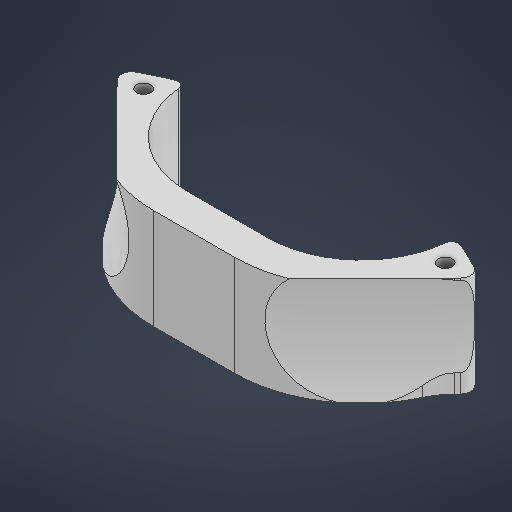
# Autodesk Inventor part: Ballkuhle
Saved by Autodesk Inventor 2025.3 (Build 293356000, 356)
## iProperties
Created: 2024-10-04
Part Number: Ballkuhle
Material: Generisch
Document SubType Name: Modeling
Designer: Mathimazierer
Density: 1 g/cm^3
Appearance: Vorgabe
Author: Mathimazierer
Autodesk Inventor part; units mm, degrees
ref_plane "YZ Plane" through (0, 0, 0) normal (1, 0, 0) x (0, 1, 0)
ref_plane "XZ Plane" through (0, 0, 0) normal (0, 1, 0) x (-1, 0, 0)
ref_plane "XY Plane" through (0, 0, 0) normal (0, 0, 1) x (1, 0, 0)
sketch "Skizze6" plane through (0, 0, 0) normal (0, 0, 1) x (1, 0, 0)
  arc A0 (21.4454, -27.1023) -> (20.0312, -26.5165) centre (20.0312, -28.5165) ccw
  line L0 (20.0312, -26.5165) -> (-20.0312, -26.5165)
  arc A1 (-20.0312, -26.5165) -> (-21.4454, -27.1023) centre (-20.0312, -28.5165) ccw
  line L1 (-21.4454, -27.1023) -> (-51.9723, -57.6292)
  line L2 (-51.9723, -57.6292) -> (-42.4264, -67.1751)
  arc A2 (-38.3776, -89.6293) -> (-42.4264, -67.1751) centre (-56.5685, -81.3173) ccw
  arc A3 (-38.3776, -89.6293) -> (38.3776, -89.6293) centre (0, 0) ccw
  arc A4 (42.4264, -67.1751) -> (38.3776, -89.6293) centre (56.5685, -81.3173) ccw
  line L3 (42.4264, -67.1751) -> (51.9724, -57.6292)
  line L4 (51.9724, -57.6292) -> (21.4454, -27.1023)
  circle A5 centre (37.8302, -37.8302) radius 1.65
  circle A6 centre (37.8302, 37.8302) radius 1.65
  circle A7 centre (-37.8302, -37.8302) radius 1.65
  circle A8 centre (-37.8302, 37.8302) radius 1.65
  circle A9 centre (-22.7665, 22.7665) radius 1.6
  circle A10 centre (22.7665, 22.7665) radius 1.6
  circle A11 centre (22.7665, -22.7665) radius 1.6
  circle A12 centre (-22.7665, -22.7665) radius 1.6
  line L5 (19.0165, -19.0165) -> (19.0165, 19.0165)
  line L6 (19.0165, 19.0165) -> (-19.0165, 19.0165)
  line L7 (-19.0165, 19.0165) -> (-19.0165, -19.0165)
  line L8 (-19.0165, -19.0165) -> (19.0165, -19.0165)
  line L9 (26.5165, -20.8596) -> (57.6292, -51.9723)
  line L10 (57.6292, -51.9723) -> (67.1751, -42.4264)
  arc A13 (89.6293, -38.3776) -> (67.1751, -42.4264) centre (81.3173, -56.5685) ccw
  arc A14 (89.6293, -38.3776) -> (89.6293, 38.3776) centre (0, 0) ccw
  arc A15 (67.1751, 42.4264) -> (89.6293, 38.3776) centre (81.3173, 56.5685) ccw
  line L11 (67.1751, 42.4264) -> (57.6292, 51.9724)
  line L12 (57.6292, 51.9724) -> (26.5165, 20.8597)
  line L13 (26.5165, 20.8597) -> (26.5165, -20.8596)
  line L14 (-26.5165, 20.8596) -> (-57.6292, 51.9723)
  line L15 (-57.6292, 51.9723) -> (-67.1751, 42.4264)
  arc A16 (-89.6293, 38.3776) -> (-67.1751, 42.4264) centre (-81.3173, 56.5685) ccw
  arc A17 (-89.6293, 38.3776) -> (-89.6293, -38.3776) centre (0, 0) ccw
  arc A18 (-67.1751, -42.4264) -> (-89.6293, -38.3776) centre (-81.3173, -56.5685) ccw
  line L16 (-67.1751, -42.4264) -> (-57.6292, -51.9724)
  line L17 (-57.6292, -51.9724) -> (-26.5165, -20.8597)
  line L18 (-26.5165, -20.8597) -> (-26.5165, 20.8596)
  circle A19 centre (-44.3776, -92.6293) radius 1.6
  circle A20 centre (92.6293, 44.3776) radius 1.6
  circle A21 centre (-92.6293, -44.3776) radius 1.6
  circle A22 centre (44.3776, -92.6293) radius 1.6
  circle A23 centre (92.6293, -44.3776) radius 1.6
  circle A24 centre (-92.6293, 44.3776) radius 1.6
  circle A25 centre (45, 91.781) radius 1.6
  circle A26 centre (-45, 91.781) radius 1.6
  circle A27 centre (-67.8822, -48.7904) radius 1.6
  circle A28 centre (-48.7904, -67.8823) radius 1.6
  circle A29 centre (48.7904, -67.8822) radius 1.6
  circle A30 centre (67.8823, -48.7904) radius 1.6
  circle A31 centre (-67.8823, 48.7904) radius 1.6
  circle A32 centre (67.8822, 48.7904) radius 1.6
  circle A33 centre (48.7904, 67.8823) radius 1.6
  circle A34 centre (-48.7904, 67.8822) radius 1.6
  arc A35 (12, 61.781) -> (38.5642, 72.6085) centre (12, 99.781) ccw
  line L19 (12, 61.781) -> (-12, 61.781)
  arc A36 (-38.5642, 72.6085) -> (-12, 61.781) centre (-12, 99.781) ccw
  arc A37 (-42.4264, 67.1751) -> (-38.5642, 72.6085) centre (-56.5685, 81.3173) ccw
  line L20 (-42.4264, 67.1751) -> (-51.9724, 57.6292)
  line L21 (-51.9724, 57.6292) -> (-20.8597, 26.5165)
  line L22 (-20.8597, 26.5165) -> (20.8596, 26.5165)
  line L23 (20.8596, 26.5165) -> (51.9723, 57.6292)
  line L24 (51.9723, 57.6292) -> (42.4264, 67.1751)
  arc A38 (38.5642, 72.6085) -> (42.4264, 67.1751) centre (56.5685, 81.3173) ccw
  line L25 (-12, 71.781) -> (12, 71.781)
  arc A39 (12, 71.781) -> (39.8653, 97.0378) centre (12, 99.781) ccw
  arc A40 (42.6492, 98.6778) -> (39.8653, 97.0378) centre (41.8557, 96.8419) ccw
  arc A41 (50.5184, 94.8902) -> (42.6492, 98.6778) centre (0, 0) ccw
  arc A42 (51.2299, 90.1207) -> (50.5184, 94.8902) centre (49.1086, 92.2421) ccw
  line L26 (51.2299, 90.1207) -> (49.4975, 88.3883)
  arc A43 (49.4975, 88.3883) -> (49.4975, 74.2462) centre (56.5685, 81.3173) ccw
  line L27 (49.4975, 74.2462) -> (74.2462, 49.4975)
  arc A44 (74.2462, 49.4975) -> (88.3884, 49.4975) centre (81.3173, 56.5685) ccw
  line L28 (88.3884, 49.4975) -> (90.1208, 51.2299)
  arc A45 (94.8902, 50.5184) -> (90.1208, 51.2299) centre (92.2421, 49.1086) ccw
  arc A46 (94.8902, -50.5184) -> (94.8902, 50.5184) centre (0, 0) ccw
  arc A47 (90.1208, -51.2299) -> (94.8902, -50.5184) centre (92.2421, -49.1086) ccw
  line L29 (90.1208, -51.2299) -> (88.3883, -49.4975)
  arc A48 (88.3883, -49.4975) -> (74.2462, -49.4975) centre (81.3173, -56.5685) ccw
  line L30 (74.2462, -49.4975) -> (49.4975, -74.2462)
  arc A49 (49.4975, -74.2462) -> (49.4975, -88.3883) centre (56.5685, -81.3173) ccw
  line L31 (49.4975, -88.3883) -> (51.2299, -90.1207)
  arc A50 (50.5184, -94.8902) -> (51.2299, -90.1207) centre (49.1086, -92.2421) ccw
  arc A51 (-50.5184, -94.8902) -> (50.5184, -94.8902) centre (0, 0) ccw
  arc A52 (-51.2299, -90.1208) -> (-50.5184, -94.8902) centre (-49.1086, -92.2421) ccw
  line L32 (-51.2299, -90.1208) -> (-49.4975, -88.3883)
  arc A53 (-49.4975, -88.3883) -> (-49.4975, -74.2462) centre (-56.5685, -81.3173) ccw
  line L33 (-49.4975, -74.2462) -> (-74.2462, -49.4975)
  arc A54 (-74.2462, -49.4975) -> (-88.3883, -49.4975) centre (-81.3173, -56.5685) ccw
  line L34 (-88.3883, -49.4975) -> (-90.1207, -51.2299)
  arc A55 (-94.8902, -50.5184) -> (-90.1207, -51.2299) centre (-92.2421, -49.1086) ccw
  arc A56 (-94.8902, 50.5184) -> (-94.8902, -50.5184) centre (0, 0) ccw
  arc A57 (-90.1208, 51.2299) -> (-94.8902, 50.5184) centre (-92.2421, 49.1086) ccw
  line L35 (-90.1208, 51.2299) -> (-88.3883, 49.4975)
  arc A58 (-88.3883, 49.4975) -> (-74.2462, 49.4975) centre (-81.3173, 56.5685) ccw
  line L36 (-74.2462, 49.4975) -> (-49.4975, 74.2462)
  arc A59 (-49.4975, 74.2462) -> (-49.4975, 88.3883) centre (-56.5685, 81.3173) ccw
  line L37 (-49.4975, 88.3883) -> (-51.2299, 90.1207)
  arc A60 (-50.5184, 94.8902) -> (-51.2299, 90.1207) centre (-49.1086, 92.2421) ccw
  arc A61 (-42.6492, 98.6778) -> (-50.5184, 94.8902) centre (0, 0) ccw
  arc A62 (-39.8653, 97.0378) -> (-42.6492, 98.6778) centre (-41.8557, 96.8419) ccw
  arc A63 (-39.8653, 97.0378) -> (-12, 71.781) centre (-12, 99.781) ccw
  arc A64 (-47.6003, 86.4911) -> (-12, 61.781) centre (-12, 99.781) ccw
  line L38 (-49.4975, 88.3883) -> (-47.6003, 86.4911)
  line L39 (0, 71.781) -> (0, 61.781) construction
  arc A65 (12, 61.781) -> (47.6003, 86.4911) centre (12, 99.781) ccw
  line L40 (49.4975, 88.3883) -> (47.6003, 86.4911)
  point P0 (0, 0)
  point P1 (0, 0)
  point P2 (38.5642, 72.6085)
  constraints: 84 point on circle, 82 end point, 66 centre point, 2 midpoint, 2 symmetric about line, 1 coincident, 1 concentric, 1 other
extrude "Extrusion4" add sketch "Skizze6" against normal blind 30 contours L19 A36 A64 L38 L37 A60 A61 A62 A63 L25 A39 A40 A41 A42 L26 L40 A65 A35
fillet "Rundung2" radius 20 2 edges at (47.6003, 86.4911, -15) (-47.6003, 86.4911, -15)
sketch "Skizze7" plane through (0, 0, 0) normal (0, 0, 1) x (1, 0, 0)
  line L0 (0, 0) -> (-29.0841, 0) construction
  line L1 (0, 0) -> (-84.8528, 84.8528)
  line L2 (-111.3693, 68.9429) -> (-68.9429, 111.3693)
  line L3 (-68.9429, 111.3693) -> (-58.3363, 100.7627)
  line L4 (-58.3363, 100.7627) -> (-100.7627, 58.3363)
  line L5 (-100.7627, 58.3363) -> (-111.3693, 68.9429)
  line L6 (-111.3693, 68.9429) -> (-58.3363, 100.7627) construction
  line L7 (-68.9429, 111.3693) -> (-100.7627, 58.3363) construction
  dimension "d19" = 45
  dimension "d20" = 120
  dimension "d21" = 60
  dimension "d22" = 15
  constraints: 16 end point, 2 midpoint, 2 parallel, 1 perpendicular
  measures "d19" angle of L1 L0
  measures "d20" distance of L0.start L1.end
  measures "d21" distance of L2.start L2.end
  measures "d22" distance of L2.end L3.end
extrude "Extrusion5" add sketch "Skizze7" against normal blind 30
sketch "Skizze8" plane through (-68.9429, 111.3693, -30) normal (-0.7071, 0.7071, 0) x (-0.7071, -0.7071, 0)
  line L0 (60, 0) -> (0, 0) projected
  line L1 (30, 0) -> (30, 17.5)
  circle A0 centre (30, 17.5) radius 30
  line L2 (0, 30) -> (60, 30) projected
  line L3 (0, 30) -> (60, 30)
  line L4 (60, 30) -> (60, 0)
  line L5 (60, 0) -> (0, 0)
  line L6 (0, 0) -> (0, 30)
  point P0 (30, 30)
  dimension "d25" = 17.5
  dimension "d26" = 60
  constraints: 10 end point, 2 parallel, 1 centre point, 1 coincident, 1 horizontal, 1 midpoint, 1 perpendicular, 1 vertical
  measures "d25" distance of L1.start L1.end
  measures "d26" diameter of A0
extrude "Extrusion6" cut sketch "Skizze8" against normal up to surface (15 mm away) contours L0 A0 L4 | L0 A0 L2 | A0 L2 L4 | L0 L6 A0 | L6 L2 A0
extrude "Extrusion7" cut sketch "Skizze8" against normal blind 100 contours A0 L0 | L0 A0 L2 | L2 A0
mirror "Spiegeln1" about plane through (0, 0, 0) normal (1, 0, 0) of "Extrusion7"
sketch "Skizze9" plane through (0, 0, 0) normal (0, 0, 1) x (1, 0, 0)
  circle A0 centre (45, 91.781) radius 1.6 projected
  circle A1 centre (45, 91.781) radius 2.1
  circle A2 centre (-45, 91.781) radius 1.6 projected
  circle A3 centre (-45, 91.781) radius 2.1
  point P0 (0, 0)
  dimension "d31" = 4.2
  dimension "d32" = 4.2
  constraints: 2 centre point, 2 coincident
  measures "d31" diameter of A1
  measures "d32" diameter of A3
extrude "Extrusion8" cut sketch "Skizze9" against normal up to surface (30 mm away) contours A0 | A1 | A2 | A3
